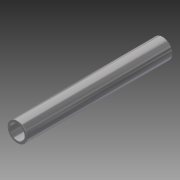
# Autodesk Inventor part: TUBE_OCG13/4x6_Open-Extend_
Saved by Autodesk Inventor 2016 SP1 (Build 200210100, 210)
## iProperties
Category: PARTsolutions
Company: PHD
Created: 2015-12-03
Part Number: TUBE_OCG13/4x6_Open-Extend_
Catalog Web Link: www.cadenas.de
Description: OCG1 Tube-OCG1 Cylinder
Vendor: PHD
Document SubType Name: Modeling
Designer: psAdmin
Manufacturer: PHD
Mass: 305.004 g
Surface Area: 260.46 cm^2
Volume: 38.1255 cm^3
Density: 8 g/cm^3
Material: Stainless Steel
Appearance: Semi-Polished
PSOL_IDENT_0: {$CADENAS_DATA\23d-libs\phd\cylinders\ocg\parts\ocg_tube.prj},266 {VTYP=3D},{NB=TUBE_OCG13/4x6_Open-
PSOL_IDENT_1: Extend_},{LINA=TUBE_OCG13/4x6_Open-Extend_},{NN=OCG1 Tube},{DATE=20.11.2015 15:31:40},{GEOMDATE=11.0
PSOL_IDENT_2: 2.2015 14:37:33},{VERSION=},{LINEID=10},{LINESUBID=-1},{WBVAR=STROKE,SWOPT,POSITION,FMTGACC,RMTGACC,
PSOL_IDENT_3: CLEVIS,HINGEPIN,SWBRKT,SWITCH}  {NB=TUBE_OCG13/4x6_Open-Extend_},{LINA=TUBE_OCG13/4x6_Open-Extend_},
PSOL_IDENT_4: {KT=DUMMY},{IDNR=OCG},{DN=1},{SIZE=3/4},{STROKE=6},{SWOPT=},{POSITION=Open-Extend},{FMTGACC=},{RMTGA
PSOL_IDENT_5: CC=},{CLEVIS=},{HINGEPIN=},{SWBRKT=},{SWITCH=},{A=0.50},{B=0.472},{D=0.24},{DD=8-32 x .28 DP},{E=1.0
PSOL_IDENT_6: 2},{EE=1/8 NPT},{H=0.16},{H1=0.44},{K=0.157},{KK=1/4-28},{LB=2.72},{MM=0.315},{N=0.94},{P=0.47},{R=0
PSOL_IDENT_7: .55},{TA=0.433},{TB=0.433},{TC=M5 X 0.8},{TD=0.315},{TE=0.157},{TF=0.020},{TG=0.217},{TR=1.54},{V=0.
PSOL_IDENT_8: 08},{W=0.50},{Y=0.97},{ZB=3.30},{ZZ=3.80},{DDDIA=0.1640},{DDDP=0.28},{KKDIA=0.2500},{TCDIA=0.1969},{
PSOL_IDENT_9: STROKE1= '1','2','3','4','5','6','7','8' },{SIZE1=0.75},{STROKE2=6},{SWOPT1= '','Blank-None','STDK2'
PSOL_IDENT_10: ,'STDK2 - DC Reed, Quick Connect','STD22','STD22 - DC Reed, 2 meter Cable','STNK2','STNK2 - DC Solid
PSOL_IDENT_11: State NPN (Sink), Quick Connect','STN22','STN22 - DC Solid State NPN (Sink), 2 meter Cable','STPK2'
PSOL_IDENT_12: ,'STPK2 - DC Solid State PNP (Source), Quick Connect','STP22','STP22 - DC Solid State PNP (Source),
PSOL_IDENT_13: 2 meter Cable' },{SWOPT2=},{OD=0.984},{LGTH=1.302},{CLEVIS1= '','Blank-None','86996-01','Rear Clevis
PSOL_IDENT_14: Hinge Mtg Kit 86996-01' },{CLEVIS2=},{PIN1= '','Blank-None' },{PIN2=},{SWBRKT1= '','Blank-None','86
PSOL_IDENT_15: 999','86999 : Round Cyl Switch Band Brkt' },{SWBRKT2=},{SWITCH1= '','Blank-None','85844-0','85844-0
PSOL_IDENT_16: : DC Reed, Quick Connect','85844-2','85844-2 : DC Reed, 2 meter Cable','85845-0','85845-0 : DC Solid
PSOL_IDENT_17: State NPN (Sink), Quick Connect','85845-2','85845-2 : DC Solid State NPN (Sink), 2 meter Cable','85
PSOL_IDENT_18: 846-0','85846-0 : DC Solid State PNP (Source), Quick Connect','85846-2','85846-2 : DC Solid State PN
PSOL_IDENT_19: P (Source), 2 meter Cable' },{SWITCH2=},{FMTGACC2=},{RMTGACC2=},{FBASE=:86993-01},{RBASE=:86993-01},
PSOL_IDENT_20: {FFLANGE=:86994-01},{RFLANGE=:86994-01},{FTRUNNION=:86995-01},{RTRUNNION=:86995-01},{FTRUNBRKT=:8699
PSOL_IDENT_21: 7-01},{RTRUNBRKT=:86997-01},{FMTGACC3=},{RMTGACC3=},{MTGACC1= '','Blank-None','86993-01','Base Mtg K
PSOL_IDENT_22: it - 86993-01','86994-01','Flange Mtg Kit - 86994-01','86995-01','Trunnion Mtg Kit - 86995-01','8699
PSOL_IDENT_23: 7-01','Hinge and Trunnion Brkt Kit - 86997-01' },{FRONTTRUNNION=0},{REARTRUNNION=0}
NN: OCG1 Tube
NT: OCG1 Cylinder
NB: TUBE_OCG13/4x6_Open-Extend_
NBSYN: TUBE_$IDNR.$DN.$SIZE.x$STROKE.$SWOPT2._$POSITION._$FMTGACC2.$RMTGACC2.$CLEVIS2.$PIN2.$SWBRKT2.$SWITCH2.
LINA: TUBE_OCG13/4x6_Open-Extend_
IDNR: OCG
DN: 1
SIZE: 3/4
STROKE: 6
SWOPT: Blank-None
POSITION: Open-Extend
FMTGACC: Blank-None
RMTGACC: Blank-None
CLEVIS: Blank-None
HINGEPIN: Blank-None
SWBRKT: Blank-None
SWITCH: Blank-None
A: 0.50
B: 0.472
D: 0.24
DD: 8-32 x .28 DP
E: 1.02
EE: 1/8 NPT
H: 0.16
H1: 0.44
K: 0.157
KK: 1/4-28
LB: 2.72
MM: 0.315
N: 0.94
P: 0.47
R: 0.55
TA: 0.433
TB: 0.433
TC: M5 X 0.8
TD: 0.315
TE: 0.157
TF: 0.020
TG: 0.217
TR: 1.54
V: 0.08
W: 0.50
Y: 0.97
ZB: 3.30
ZZ: 3.80
DDDIA: 0.1640
DDDP: 0.28
KKDIA: 0.2500
TCDIA: 0.1969
OD: 0.984
LGTH: 1.302
FBASE: :86993-01
RBASE: :86993-01
FFLANGE: :86994-01
RFLANGE: :86994-01
FTRUNNION: :86995-01
RTRUNNION: :86995-01
FTRUNBRKT: :86997-01
RTRUNBRKT: :86997-01
SUPPLIER: PHD
ARTICLENO: TUBE_OCG13/4x6_Open-Extend_
BOMINFO: TUBE_OCG13/4x6_Open-Extend_
CREATOR: CADENAS GmbH
Title: TUBE_OCG13/4x6_Open-Extend_
Author: Cadenas PARTsolutions
Comments: OCG1 Cylinder
Autodesk Inventor part; units mm, degrees
sketch "Sketch_2" plane through (0, 0, 0) normal (1, 0, 0) x (0, 1, 0)
  line L0 (0, -92.7354) -> (0, 92.7354)
  line L1 (9.525, 92.7354) -> (9.525, -92.7354)
  line L2 (9.525, -92.7354) -> (12.192, -92.7354)
  line L3 (12.192, -92.7354) -> (12.4968, -92.4306)
  line L4 (12.4968, -92.4306) -> (12.4968, 92.4306)
  line L5 (12.4968, 92.4306) -> (12.192, 92.7354)
  line L6 (12.192, 92.7354) -> (9.525, 92.7354)
  constraints: 14 end point
revolve "Revolution1" add sketch "Sketch_2" angle 360 about axis through (0, 0, -92.7354) along (0, 0, -1)
ref_plane "cap_XY" through (0, 0, -92.7354) normal (0, 0, -1) x (0, 1, 0)
ref_plane "cap_YZ" through (0, 0, -92.7354) normal (0, 1, 0) x (1, 0, 0)
ref_plane "cap_ZX" through (0, 0, -92.7354) normal (1, 0, 0) x (0, 0, -1)
ref_plane "ctr_XY" through (0, 0, 0) normal (0, 0, 1) x (1, 0, 0)
ref_plane "ctr_YZ" through (0, 0, 0) normal (1, 0, 0) x (0, 1, 0)
ref_plane "ctr_ZX" through (0, 0, 0) normal (0, 1, 0) x (0, 0, 1)
ref_plane "hd_XY" through (0, 0, 92.7354) normal (0, 0, 1) x (0, 1, 0)
ref_plane "hd_YZ" through (0, 0, 92.7354) normal (0, 1, 0) x (-1, 0, 0)
ref_plane "hd_ZX" through (0, 0, 92.7354) normal (-1, 0, 0) x (0, 0, 1)
body "Solid1"
